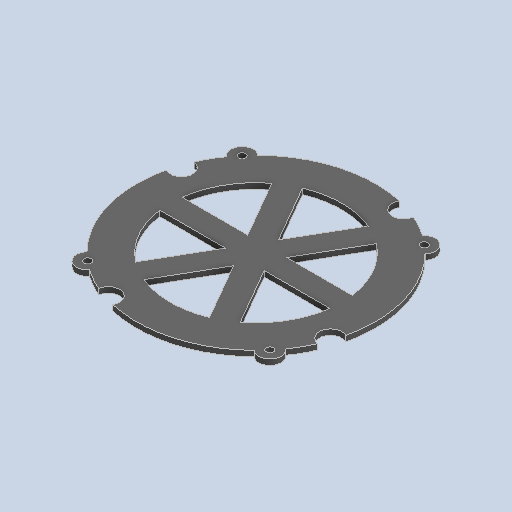
# Autodesk Inventor part: battery_cover
Saved by Autodesk Inventor 2024.1 (Build 281209000, 209)
## iProperties
Created: 2024-08-02
Part Number: battery_cover
Material: 一般
Document SubType Name: Modeling
Designer: hibik
Density: 1 g/cm^3
Appearance: 既定
Author: hibik
Autodesk Inventor part; units mm, degrees
ref_plane "YZ Plane" through (0, 0, 0) normal (1, 0, 0) x (0, 1, 0)
ref_plane "XZ Plane" through (0, 0, 0) normal (0, 1, 0) x (-1, 0, 0)
ref_plane "XY Plane" through (0, 0, 0) normal (0, 0, 1) x (1, 0, 0)
sketch "スケッチ1" plane through (0, 0, 0) normal (0, 1, 0) x (-1, 0, 0)
  circle A0 centre (0, 0) radius 42.5
  dimension "d0" = 85
  constraints: 1 centre point, 1 coincident
  measures "d0" diameter of A0
extrude "押し出し1" add sketch "スケッチ1" along normal blind 2
sketch "スケッチ2" plane through (0, 0, 0) normal (0, -1, 0) x (1, 0, 0)
  circle A0 centre (-27.4257, 32.3702) radius 1.3 projected
  circle A1 centre (32.3702, 27.4257) radius 1.3 projected
  circle A2 centre (27.4257, -32.3702) radius 1.3 projected
  circle A3 centre (-32.3702, -27.4257) radius 1.3 projected
  circle A4 centre (-32.3702, -27.4257) radius 4
  circle A5 centre (-27.4257, 32.3702) radius 4
  circle A6 centre (27.4257, -32.3702) radius 4
  circle A7 centre (32.3702, 27.4257) radius 4
  circle A8 centre (-13, 39.5) radius 1.35 projected
  circle A9 centre (39.5, 13) radius 1.35 projected
  circle A10 centre (13, -39.5) radius 1.35 projected
  circle A11 centre (-39.5, -13) radius 1.35 projected
  circle A12 centre (-39.5, -13) radius 4
  circle A13 centre (-13, 39.5) radius 4
  circle A14 centre (39.5, 13) radius 4
  circle A15 centre (13, -39.5) radius 4
  line L0 (17.7859, 38.8061) -> (-24.7141, -34.8061)
  line L1 (-24.7141, -34.8061) -> (-17.7859, -38.8061)
  line L2 (-17.7859, -38.8061) -> (24.7141, 34.8061)
  line L3 (24.7141, 34.8061) -> (17.7859, 38.8061)
  line L4 (17.7859, 38.8061) -> (-17.7859, -38.8061) construction
  line L5 (-24.7141, -34.8061) -> (24.7141, 34.8061) construction
  line L6 (17.7859, -38.8061) -> (-24.7141, 34.8061)
  line L7 (-24.7141, 34.8061) -> (-17.7859, 38.8061)
  line L8 (-17.7859, 38.8061) -> (24.7141, -34.8061)
  line L9 (24.7141, -34.8061) -> (17.7859, -38.8061)
  line L10 (17.7859, -38.8061) -> (-17.7859, 38.8061) construction
  line L11 (-24.7141, 34.8061) -> (24.7141, -34.8061) construction
  line L12 (42.5, -4) -> (-42.5, -4)
  line L13 (-42.5, -4) -> (-42.5, 4)
  line L14 (-42.5, 4) -> (42.5, 4)
  line L15 (42.5, 4) -> (42.5, -4)
  line L16 (42.5, -4) -> (-42.5, 4) construction
  line L17 (-42.5, -4) -> (42.5, 4) construction
  line L18 (-42.5, 24.5374) -> (0, 49.0748) construction
  line L19 (0, 49.0748) -> (42.5, 24.5374) construction
  line L20 (42.5, 24.5374) -> (42.5, -24.5374) construction
  line L21 (42.5, -24.5374) -> (0, -49.0748) construction
  line L22 (0, -49.0748) -> (-42.5, -24.5374) construction
  line L23 (-42.5, -24.5374) -> (-42.5, 24.5374) construction
  circle A16 centre (0, 0) radius 42.5 projected
  circle A17 centre (0, 0) radius 30.5
  point P0 (-11.6542, -28.1856)
  point P1 (11.6542, -28.1856)
  point P2 (0, -8)
  point P3 (18.5824, -24.1856)
  point P4 (30.2366, -4)
  point P5 (6.9282, -4)
  point P6 (30.2366, 4)
  point P7 (18.5824, 24.1856)
  point P8 (6.9282, 4)
  point P9 (11.6542, 28.1856)
  point P10 (-11.6542, 28.1856)
  point P11 (0, 8)
  point P12 (-18.5824, 24.1856)
  point P13 (-30.2366, 4)
  point P14 (-6.9282, 4)
  point P15 (-30.2366, -4)
  point P16 (-18.5824, -24.1856)
  point P17 (-6.9282, -4)
  point P18 (-26.4694, 33.2509)
  point P19 (-28.4514, 31.5716)
  point P20 (-33.2509, -26.4694)
  point P21 (-31.5716, -28.4514)
  dimension "d3" = 8
  dimension "d6" = 8
  dimension "d7" = 12
  constraints: 48 end point, 10 coincident, 9 centre point, 7 equal radius, 6 midpoint, 6 parallel, 3 collinear, 3 perpendicular, 2 equal length, 1 horizontal, 1 tangent, 1 vertical, 13 other
  measures "d3" diameter of A4
  measures "d6" distance between parallel lines of L14 L12
  measures "d7" radial gap between concentric circles of A16 A17
extrude "押し出し2" cut sketch "スケッチ2" against normal through all contours A0 A16 | L6 L14 A17 | A17 L0 L8 | L12 L0 A17 | A16 A8 A13 | A13 A16 A8 | A16 A11 A12 | A12 A16 A11 | A17 L14 L2 | A16 A8 | A8 A16 | L2 L6 A17 | A16 A11 | A11 A16 | L12 A17 L8 | A16 A3 | A16 A10 A15 | A15 A16 A10 | A16 A1 | A1 A16 | A16 A9 A14 | A14 A16 A9 | A16 A10 | A10 A16 | A16 A9 | A9 A16 | A16 A2 | A2 A16 picked at (-27.1376, 32.113) picked at (-32.0736, -27.1791)
sketch "スケッチ3" plane through (0, 0, 0) normal (0, -1, 0) x (1, 0, 0)
  arc A0 (-31.5716, -28.4514) -> (-33.2509, -26.4694) centre (-32.3702, -27.4257) ccw projected
  arc A1 (-28.4514, 31.5716) -> (-26.4694, 33.2509) centre (-27.4257, 32.3702) ccw projected
  arc A2 (31.5716, 28.4514) -> (33.2509, 26.4694) centre (32.3702, 27.4257) ccw projected
  arc A3 (28.4514, -31.5716) -> (26.4694, -33.2509) centre (27.4257, -32.3702) ccw projected
  circle A4 centre (-32.3702, -27.4257) radius 1.3
  circle A5 centre (-27.4257, 32.3702) radius 1.3
  circle A6 centre (32.3702, 27.4257) radius 1.3
  circle A7 centre (27.4257, -32.3702) radius 1.3
  circle A8 centre (-32.3702, -27.4257) radius 4
  circle A9 centre (-27.4257, 32.3702) radius 4
  circle A10 centre (32.3702, 27.4257) radius 4
  circle A11 centre (27.4257, -32.3702) radius 4
  point P0 (0, 0)
  point P1 (28.4514, -31.5716)
  point P2 (-26.4694, 33.2509)
  dimension "d10" = 8
  constraints: 8 centre point, 8 coincident, 7 equal radius
  measures "d10" diameter of A8
ref_plane "作業平面1" through (-124.0859, 3.5, -124.0859) normal (0, 1, 0) x (0.0824091, 0, 0.9965986)
extrude "押し出し3" add sketch "スケッチ3" against normal up to surface (2 mm away)
